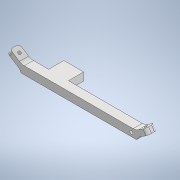
# Autodesk Inventor part: leg_switch_holder_1
Saved by Autodesk Inventor 2020 (Build 240168000, 168)
## iProperties
Created: 2019-08-05
Part Number: leg_switch_holder_1
Material: Generic
Document SubType Name: Modeling
Designer: psrob
Density: 1 g/cm^3
Appearance: Default
Author: psrob
Autodesk Inventor part; units mm, degrees
ref_plane "YZ Plane" through (0, 0, 0) normal (1, 0, 0) x (0, 1, 0)
ref_plane "XZ Plane" through (0, 0, 0) normal (0, 1, 0) x (-1, 0, 0)
ref_plane "XY Plane" through (0, 0, 0) normal (0, 0, 1) x (1, 0, 0)
sketch "Sketch1" plane through (0, 0, 0) normal (0, 0, 1) x (1, 0, 0)
  line L0 (96, 6.7) -> (90, 2.7) projected
  line L1 (10, 2.5) -> (2, 7.5) projected
  line L2 (0, 0) -> (100, 0) projected
  line L3 (96, 6.7) -> (96, 10.7) projected
  line L4 (2, 7.5) -> (3.855, 10.468)
  line L5 (96, 6.7) -> (94.0585, 9.6122)
  line L6 (94.0585, 9.6122) -> (87.4021, 5.1746)
  line L7 (3.855, 10.468) -> (12.3391, 5.1746)
  line L8 (87.4021, 5.1746) -> (12.3391, 5.1746)
  line L9 (90, 2.7) -> (88.3359, 1.5906)
  line L10 (88.3359, 1.5906) -> (88.3359, 0)
  line L11 (10, 2.5) -> (11.696, 1.44)
  line L12 (11.696, 1.44) -> (11.696, 0)
  line L13 (88.3359, 0) -> (11.696, 0)
  dimension "d0" = 3.5
  dimension "d1" = 3.5
  dimension "d2" = 8
  dimension "d3" = 10
  dimension "d4" = 2
  dimension "d5" = 2
  constraints: 20 end point, 3 collinear, 3 perpendicular, 2 point on line, 1 horizontal
  measures "d0" distance of L1.end L4.end
  measures "d1" distance of L0.start L5.end
  measures "d2" distance of L5.end L6.end
  measures "d3" distance of L4.end L7.end
  measures "d4" distance of L0.end L9.end
  measures "d5" distance of L1.start L11.end
ref_plane "Work Plane1" through (0, -6, -6) normal (0, 0, -1) x (0, 1, 0)
extrude "Extrusion1" add sketch "Sketch1" against normal up to surface (6 mm away)
sketch "Sketch2" plane through (87.4021, 5.1746, 0) normal (-0.5547002, 0.8320503, 0) x (0.8320503, 0.5547002, 0)
  circle A0 centre (4.3944, 3) radius 1 projected
  point P0 (-75.5933, 0)
extrude "Extrusion2" cut sketch "Sketch2" against normal blind 10
sketch "Sketch3" plane through (3.855, 10.468, 0) normal (0.529342, 0.8484086, 0) x (0.8484086, -0.529342, 0)
  ellipse E0 centre (4.7143, 3) end of major axis (4.7143, 2) minor radius 1 projected
  point P0 (2.2705, 0)
extrude "Extrusion3" cut sketch "Sketch3" against normal blind 10
fillet "Fillet1" radius 2 2 edges at (2.9275, 8.984, 0) (2.9275, 8.984, -6)
thicken "Thicken1" operation add thickness 1 both sides no extend neighbours yes toward (0.8479983, -0.5299989, 0) faces at (3.2367, 9.4787, -3.3333)
fillet "Fillet2" radius 2 2 edges at (95.0293, 8.1561, 0) (95.0293, 8.1561, -6)
thicken "Thicken2" operation add thickness 0.5 both sides no extend neighbours yes toward (-0.8320503, -0.5547002, 0) faces at (95.3528, 7.6707, -3.3333)
fillet "Fillet3" radius 6 2 edges at (87.4021, 5.1746, -3) (12.3391, 5.1746, -3)
fillet "Fillet4" radius 3 2 edges at (88.3359, 1.5906, -3) (11.696, 1.44, -3)
sketch "Sketch4" plane through (0, 0, 0) normal (0, 0, 1) x (1, 0, 0)
  ellipse E0 centre (138.3197, 3) end of major axis (138.3197, 2.6) minor radius 0.3168 (138.0029, 3) -> (138.3197, 3.4) ccw projected
  line L0 (138.3197, 3.4) -> (141.963, 3.4) projected
  line L1 (141.963, 3.4) -> (141.963, 4.4) projected
  line L2 (141.963, 4.4) -> (132.2441, 4.4) projected
  line L3 (132.2441, 1.4) -> (132.2441, 4.4) projected
  line L4 (141.963, 1.4) -> (132.2441, 1.4) projected
  line L5 (141.963, 1.4) -> (141.963, 2.4) projected
  line L6 (141.963, 2.4) -> (138.0029, 2.4) projected
  ellipse E1 centre (138.3197, 2.8) end of major axis (138.3197, 2.4) minor radius 0.3168 (138.0029, 2.8) -> (138.0029, 2.8) ccw projected
  line L7 (138.0029, 2.8) -> (138.0029, 3) projected
  line L8 (91.9784, 8.2254) -> (93.9199, 5.3132) projected
  line L9 (91.9784, 8.2254) -> (88.9137, 6.1823) projected
  arc A0 (85.5855, 5.1746) -> (88.9137, 6.1823) centre (85.5855, 11.1746) ccw projected
  line L10 (85.5855, 5.1746) -> (14.0573, 5.1746) projected
  arc A1 (10.8813, 6.0841) -> (14.0573, 5.1746) centre (14.0573, 11.1746) ccw projected
  line L11 (10.8813, 6.0841) -> (6.4002, 8.88) projected
  line L12 (4.544, 5.91) -> (6.4002, 8.88) projected
  line L13 (4.544, 5.91) -> (10.2947, 2.3158) projected
  arc A2 (11.696, 0) -> (10.2947, 2.3158) centre (8.7047, -0.2282) ccw projected
  line L14 (11.696, 0) -> (88.3359, 0) projected
  arc A3 (89.6718, 2.4812) -> (88.3359, 0) centre (91.3359, -0.015) ccw projected
  line L15 (89.6718, 2.4812) -> (93.9199, 5.3132) projected
  line L16 (88.3359, 0) -> (84.3359, 0)
  line L17 (11.696, 0) -> (88.3359, 0) projected
  line L18 (84.3359, 0) -> (81.3359, 0)
  line L19 (84.3359, 0) -> (84.3359, 2.5)
  line L20 (85.5855, 5.1746) -> (14.0573, 5.1746) projected
  circle A4 centre (84.3359, 2.5) radius 1
  point P0 (0, 0)
  dimension "d20" = 4
  dimension "d21" = 3
  dimension "d22" = 2.5
  dimension "d23" = 2
  constraints: 6 end point, 2 point on line, 1 centre point, 1 coincident, 1 perpendicular, 3 other
  measures "d20" distance of L14.end L16.end
  measures "d21" distance of L16.end L18.end
  measures "d22" distance of L16.end L19.end
  measures "d23" diameter of A4
extrude "Extrusion4" cut sketch "Sketch4" against normal blind 10 contours A4
fillet "Fillet5" radius 1 2 edges at (88.3359, 0, -3) (11.6877, 0, -3)
sketch "Sketch5" plane through (14.0573, 5.1746, 0) normal (0, 1, 0) x (1, 0, 0)
  line L0 (0, 0) -> (0, 6) projected
  line L1 (71.5281, 0) -> (0, 0) projected
  line L2 (71.5281, 6) -> (71.5281, 0) projected
  line L3 (71.5281, 6) -> (0, 6) projected
  line L4 (0, 6) -> (0, 6)
  line L5 (-1.5459, 6) -> (73.4094, 6) projected
  line L6 (0, 6) -> (13, 6)
  line L7 (13, 6) -> (13, 16)
  line L8 (13, 16) -> (0, 16)
  line L9 (0, 16) -> (0, 6)
  point P0 (-14.0573, 0)
  dimension "d27" = 0
  dimension "d28" = 13
  dimension "d29" = 10
  constraints: 10 end point, 2 parallel, 1 horizontal, 1 perpendicular, 1 point on line
  measures "d27" distance of L0.end L4.end
  measures "d28" distance of L8.end L7.end
  measures "d29" distance of L7.end L6.end
extrude "Extrusion5" add sketch "Sketch5" against normal up to surface (5.1746 mm away) contours L9 L8 L7 L3
sketch "Sketch6" plane through (14.0573, 5.1746, 0) normal (0, 1, 0) x (1, 0, 0)
  line L0 (0, 0) -> (0, 6) projected
  line L1 (71.5281, 0) -> (0, 0) projected
  line L2 (71.5281, 6) -> (71.5281, 0) projected
  line L3 (71.5281, 6) -> (13, 6) projected
  line L4 (13, 6) -> (13, 16) projected
  line L5 (13, 16) -> (0, 16) projected
  line L6 (0, 16) -> (0, 6) projected
  line L7 (13, 6) -> (-10, 6)
  point P0 (-14.0573, 0)
  constraints: 2 end point, 1 horizontal
extrude "Extrusion6" cut sketch "Sketch6" against normal blind 2 contours L6 L5 L4 L7
body "Solid1"
